Autodesk Inventor part; units mm, degrees
(part 3 of 4)
  spline S285 degree 2 poles (-3.3011, -25.9949) (-3.1963, -25.928) (-3.0357, -25.8098) knots 0 0 0 1 1 1
  line L1033 (-3.3011, -25.9949) -> (-3.1963, -25.928) construction
  line L1034 (-3.1963, -25.928) -> (-3.0357, -25.8098) construction
  spline S286 degree 2 poles (-3.0357, -25.8098) (-2.8751, -25.6805) (-2.8751, -25.5801) knots 0 0 0 1 1 1
  line L1035 (-3.0357, -25.8098) -> (-2.8751, -25.6805) construction
  line L1036 (-2.8751, -25.6805) -> (-2.8751, -25.5801) construction
  spline S287 degree 2 poles (-2.8751, -25.5801) (-2.8751, -25.4775) (-2.942, -25.4195) knots 0 0 0 1 1 1
  line L1037 (-2.8751, -25.5801) -> (-2.8751, -25.4775) construction
  line L1038 (-2.8751, -25.4775) -> (-2.942, -25.4195) construction
  spline S288 degree 2 poles (-2.942, -25.4195) (-3.0022, -25.3682) (-3.087, -25.3682) knots 0 0 0 1 1 1
  line L1039 (-2.942, -25.4195) -> (-3.0022, -25.3682) construction
  line L1040 (-3.0022, -25.3682) -> (-3.087, -25.3682) construction
  spline S289 degree 2 poles (-3.087, -25.3682) (-3.1762, -25.3682) (-3.2342, -25.4195) knots 0 0 0 1 1 1
  line L1041 (-3.087, -25.3682) -> (-3.1762, -25.3682) construction
  line L1042 (-3.1762, -25.3682) -> (-3.2342, -25.4195) construction
  spline S290 degree 2 poles (-3.2342, -25.4195) (-3.3011, -25.4775) (-3.3011, -25.5801) knots 0 0 0 1 1 1
  line L1043 (-3.2342, -25.4195) -> (-3.3011, -25.4775) construction
  line L1044 (-3.3011, -25.4775) -> (-3.3011, -25.5801) construction
  spline S291 degree 2 poles (-2.768, -27.5026) (-2.6588, -27.5026) (-2.5026, -27.3443) (-2.5026, -27.235) knots 0 0 0 1 2 2 2
  line L1045 (-2.768, -27.5026) -> (-2.6588, -27.5026) construction
  line L1046 (-2.6588, -27.5026) -> (-2.5026, -27.3443) construction
  line L1047 (-2.5026, -27.3443) -> (-2.5026, -27.235) construction
  line L1048 (-2.5026, -27.235) -> (-2.5026, -26.4343)
  spline S292 degree 2 poles (-2.5026, -26.4343) (-2.5026, -26.325) (-2.6588, -26.1667) (-2.768, -26.1667) knots 0 0 0 1 2 2 2
  line L1049 (-2.5026, -26.4343) -> (-2.5026, -26.325) construction
  line L1050 (-2.5026, -26.325) -> (-2.6588, -26.1667) construction
  line L1051 (-2.6588, -26.1667) -> (-2.768, -26.1667) construction
  line L1052 (-2.768, -26.1667) -> (-3.0357, -26.1667)
  spline S293 degree 2 poles (-3.0357, -26.1667) (-3.145, -26.1667) (-3.3011, -26.325) (-3.3011, -26.4343) knots 0 0 0 1 2 2 2
  line L1053 (-3.0357, -26.1667) -> (-3.145, -26.1667) construction
  line L1054 (-3.145, -26.1667) -> (-3.3011, -26.325) construction
  line L1055 (-3.3011, -26.325) -> (-3.3011, -26.4343) construction
  line L1056 (-3.3011, -26.4343) -> (-3.3011, -27.235)
  spline S294 degree 2 poles (-3.3011, -27.235) (-3.3011, -27.3443) (-3.145, -27.5026) (-3.0357, -27.5026) knots 0 0 0 1 2 2 2
  line L1057 (-3.3011, -27.235) -> (-3.3011, -27.3443) construction
  line L1058 (-3.3011, -27.3443) -> (-3.145, -27.5026) construction
  line L1059 (-3.145, -27.5026) -> (-3.0357, -27.5026) construction
  line L1060 (-3.0357, -27.5026) -> (-2.768, -27.5026)
  spline S295 degree 2 poles (-2.3666, -26.0619) (-2.235, -26.2024) (-2.235, -26.4343) knots 0 0 0 1 1 1
  line L1061 (-2.3666, -26.0619) -> (-2.235, -26.2024) construction
  line L1062 (-2.235, -26.2024) -> (-2.235, -26.4343) construction
  line L1063 (-2.235, -26.4343) -> (-2.235, -27.2372)
  spline S296 degree 2 poles (-2.235, -27.2372) (-2.235, -27.458) (-2.5472, -27.7703) (-2.768, -27.7703) knots 0 0 0 1 2 2 2
  line L1064 (-2.235, -27.2372) -> (-2.235, -27.458) construction
  line L1065 (-2.235, -27.458) -> (-2.5472, -27.7703) construction
  line L1066 (-2.5472, -27.7703) -> (-2.768, -27.7703) construction
  line L1067 (-2.768, -27.7703) -> (-3.0357, -27.7703)
  spline S297 degree 2 poles (-3.0357, -27.7703) (-3.2542, -27.7703) (-3.5687, -27.458) (-3.5687, -27.2372) knots 0 0 0 1 2 2 2
  line L1068 (-3.0357, -27.7703) -> (-3.2542, -27.7703) construction
  line L1069 (-3.2542, -27.7703) -> (-3.5687, -27.458) construction
  line L1070 (-3.5687, -27.458) -> (-3.5687, -27.2372) construction
  line L1071 (-3.5687, -27.2372) -> (-3.5687, -25.5801)
  spline S298 degree 2 poles (-3.5687, -25.5801) (-3.5687, -25.3549) (-3.4193, -25.221) knots 0 0 0 1 1 1
  line L1072 (-3.5687, -25.5801) -> (-3.5687, -25.3549) construction
  line L1073 (-3.5687, -25.3549) -> (-3.4193, -25.221) construction
  spline S299 degree 2 poles (-3.4193, -25.221) (-3.2832, -25.1006) (-3.0847, -25.1006) knots 0 0 0 1 1 1
  line L1074 (-3.4193, -25.221) -> (-3.2832, -25.1006) construction
  line L1075 (-3.2832, -25.1006) -> (-3.0847, -25.1006) construction
  spline S300 degree 2 poles (-3.0847, -25.1006) (-2.8907, -25.1006) (-2.7569, -25.2188) knots 0 0 0 1 1 1
  line L1076 (-3.0847, -25.1006) -> (-2.8907, -25.1006) construction
  line L1077 (-2.8907, -25.1006) -> (-2.7569, -25.2188) construction
  spline S301 degree 2 poles (-2.7569, -25.2188) (-2.6075, -25.3526) (-2.6075, -25.5779) knots 0 0 0 1 1 1
  line L1078 (-2.7569, -25.2188) -> (-2.6075, -25.3526) construction
  line L1079 (-2.6075, -25.3526) -> (-2.6075, -25.5779) construction
  spline S302 degree 2 poles (-2.6075, -25.5779) (-2.6075, -25.8031) (-2.768, -25.9102) knots 0 0 0 1 1 1
  line L1080 (-2.6075, -25.5779) -> (-2.6075, -25.8031) construction
  line L1081 (-2.6075, -25.8031) -> (-2.768, -25.9102) construction
  spline S303 degree 2 poles (-2.768, -25.9102) (-2.5093, -25.9102) (-2.3666, -26.0619) knots 0 0 0 1 1 1
  line L1082 (-2.768, -25.9102) -> (-2.5093, -25.9102) construction
  line L1083 (-2.5093, -25.9102) -> (-2.3666, -26.0619) construction
  spline S304 degree 2 poles (0.7023, -26.1689) (0.5774, -26.1689) (0.4369, -26.325) (0.4369, -26.4343) knots 0 0 0 1 2 2 2
  line L1084 (0.7023, -26.1689) -> (0.5774, -26.1689) construction
  line L1085 (0.5774, -26.1689) -> (0.4369, -26.325) construction
  line L1086 (0.4369, -26.325) -> (0.4369, -26.4343) construction
  spline S305 degree 2 poles (0.4369, -26.4343) (0.4369, -26.5436) (0.5038, -26.6194) knots 0 0 0 1 1 1
  line L1087 (0.4369, -26.4343) -> (0.4369, -26.5436) construction
  line L1088 (0.4369, -26.5436) -> (0.5038, -26.6194) construction
  spline S306 degree 2 poles (0.5038, -26.6194) (0.5774, -26.7019) (0.7023, -26.7019) knots 0 0 0 1 1 1
  line L1089 (0.5038, -26.6194) -> (0.5774, -26.7019) construction
  line L1090 (0.5774, -26.7019) -> (0.7023, -26.7019) construction
  spline S307 degree 2 poles (0.4146, -27.71) (0.3744, -27.7725) (0.3075, -27.7725) knots 0 0 0 1 1 1
  line L1091 (0.4146, -27.71) -> (0.3744, -27.7725) construction
  line L1092 (0.3744, -27.7725) -> (0.3075, -27.7725) construction
  spline S308 degree 2 poles (0.3075, -27.7725) (0.2518, -27.7725) (0.167, -27.6922) (0.167, -27.6387) knots 0 0 0 1 2 2 2
  line L1093 (0.3075, -27.7725) -> (0.2518, -27.7725) construction
  line L1094 (0.2518, -27.7725) -> (0.167, -27.6922) construction
  line L1095 (0.167, -27.6922) -> (0.167, -27.6387) construction
  spline S309 degree 2 poles (0.167, -27.6387) (0.167, -27.5985) (0.1916, -27.5628) knots 0 0 0 1 1 1
  line L1096 (0.167, -27.6387) -> (0.167, -27.5985) construction
  line L1097 (0.167, -27.5985) -> (0.1916, -27.5628) construction
  line L1098 (0.1916, -27.5628) -> (0.593, -26.9607)
  spline S310 degree 2 poles (0.593, -26.9607) (0.3923, -26.9272) (0.2741, -26.7689) knots 0 0 0 1 1 1
  line L1099 (0.593, -26.9607) -> (0.3923, -26.9272) construction
  line L1100 (0.3923, -26.9272) -> (0.2741, -26.7689) construction
  spline S311 degree 2 poles (0.2741, -26.7689) (0.1692, -26.6261) (0.1692, -26.4343) knots 0 0 0 1 1 1
  line L1101 (0.2741, -26.7689) -> (0.1692, -26.6261) construction
  line L1102 (0.1692, -26.6261) -> (0.1692, -26.4343) construction
  spline S312 degree 2 poles (0.1692, -26.4343) (0.1692, -26.218) (0.3031, -26.0685) knots 0 0 0 1 1 1
  line L1103 (0.1692, -26.4343) -> (0.1692, -26.218) construction
  line L1104 (0.1692, -26.218) -> (0.3031, -26.0685) construction
  spline S313 degree 2 poles (0.3031, -26.0685) (0.4503, -25.9013) (0.7023, -25.9013) knots 0 0 0 1 1 1
  line L1105 (0.3031, -26.0685) -> (0.4503, -25.9013) construction
  line L1106 (0.4503, -25.9013) -> (0.7023, -25.9013) construction
  line L1107 (0.7023, -25.9013) -> (1.3691, -25.9013)
  spline S314 degree 2 poles (1.3691, -25.9013) (1.503, -25.9013) (1.503, -26.0351) knots 0 0 0 1 1 1
  line L1108 (1.3691, -25.9013) -> (1.503, -25.9013) construction
  line L1109 (1.503, -25.9013) -> (1.503, -26.0351) construction
  line L1110 (1.503, -26.0351) -> (1.503, -27.6364)
  spline S315 degree 2 poles (1.503, -27.6364) (1.503, -27.7703) (1.3691, -27.7703) knots 0 0 0 1 1 1
  line L1111 (1.503, -27.6364) -> (1.503, -27.7703) construction
  line L1112 (1.503, -27.7703) -> (1.3691, -27.7703) construction
  spline S316 degree 2 poles (1.3691, -27.7703) (1.2353, -27.7703) (1.2353, -27.6364) knots 0 0 0 1 1 1
  line L1113 (1.3691, -27.7703) -> (1.2353, -27.7703) construction
  line L1114 (1.2353, -27.7703) -> (1.2353, -27.6364) construction
  spline S317 degree 2 poles (3.1846, -27.5026) (3.2627, -27.5026) (3.3719, -27.3933) (3.3719, -27.3153) knots 0 0 0 1 2 2 2
  line L1115 (3.1846, -27.5026) -> (3.2627, -27.5026) construction
  line L1116 (3.2627, -27.5026) -> (3.3719, -27.3933) construction
  line L1117 (3.3719, -27.3933) -> (3.3719, -27.3153) construction
  line L1118 (3.3719, -27.3153) -> (3.3719, -26.3563)
  spline S318 degree 2 poles (3.3719, -26.3563) (3.3719, -26.2782) (3.2627, -26.1689) (3.1846, -26.1689) knots 0 0 0 1 2 2 2
  line L1119 (3.3719, -26.3563) -> (3.3719, -26.2782) construction
  line L1120 (3.3719, -26.2782) -> (3.2627, -26.1689) construction
  line L1121 (3.2627, -26.1689) -> (3.1846, -26.1689) construction
  line L1122 (3.1846, -26.1689) -> (3.0262, -26.1689)
  spline S319 degree 2 poles (3.0262, -26.1689) (2.9482, -26.1689) (2.8389, -26.2804) (2.8389, -26.3563) knots 0 0 0 1 2 2 2
  line L1123 (3.0262, -26.1689) -> (2.9482, -26.1689) construction
  line L1124 (2.9482, -26.1689) -> (2.8389, -26.2804) construction
  line L1125 (2.8389, -26.2804) -> (2.8389, -26.3563) construction
  line L1126 (2.8389, -26.3563) -> (2.8389, -27.3153)
  spline S320 degree 2 poles (2.8389, -27.3153) (2.8389, -27.3933) (2.9482, -27.5026) (3.0262, -27.5026) knots 0 0 0 1 2 2 2
  line L1127 (2.8389, -27.3153) -> (2.8389, -27.3933) construction
  line L1128 (2.8389, -27.3933) -> (2.9482, -27.5026) construction
  line L1129 (2.9482, -27.5026) -> (3.0262, -27.5026) construction
  line L1130 (3.0262, -27.5026) -> (3.1846, -27.5026)
  spline S321 degree 2 poles (2.5713, -26.354) (2.5713, -26.1689) (2.8367, -25.9013) (3.0262, -25.9013) knots 0 0 0 1 2 2 2
  line L1131 (2.5713, -26.354) -> (2.5713, -26.1689) construction
  line L1132 (2.5713, -26.1689) -> (2.8367, -25.9013) construction
  line L1133 (2.8367, -25.9013) -> (3.0262, -25.9013) construction
  line L1134 (3.0262, -25.9013) -> (3.1846, -25.9013)
  spline S322 degree 2 poles (3.1846, -25.9013) (3.3742, -25.9013) (3.6396, -26.1667) (3.6396, -26.3563) knots 0 0 0 1 2 2 2
  line L1135 (3.1846, -25.9013) -> (3.3742, -25.9013) construction
  line L1136 (3.3742, -25.9013) -> (3.6396, -26.1667) construction
  line L1137 (3.6396, -26.1667) -> (3.6396, -26.3563) construction
  line L1138 (3.6396, -26.3563) -> (3.6396, -27.3153)
  spline S323 degree 2 poles (3.6396, -27.3153) (3.6396, -27.5049) (3.3742, -27.7703) (3.1846, -27.7703) knots 0 0 0 1 2 2 2
  line L1139 (3.6396, -27.3153) -> (3.6396, -27.5049) construction
  line L1140 (3.6396, -27.5049) -> (3.3742, -27.7703) construction
  line L1141 (3.3742, -27.7703) -> (3.1846, -27.7703) construction
  line L1142 (3.1846, -27.7703) -> (3.0262, -27.7703)
  spline S324 degree 2 poles (3.0262, -27.7703) (2.8367, -27.7703) (2.5713, -27.5071) (2.5713, -27.3175) knots 0 0 0 1 2 2 2
  line L1143 (3.0262, -27.7703) -> (2.8367, -27.7703) construction
  line L1144 (2.8367, -27.7703) -> (2.5713, -27.5071) construction
  line L1145 (2.5713, -27.5071) -> (2.5713, -27.3175) construction
  spline S325 degree 2 poles (2.3059, -27.6364) (2.3059, -27.7703) (2.172, -27.7703) knots 0 0 0 1 1 1
  line L1146 (2.3059, -27.6364) -> (2.3059, -27.7703) construction
  line L1147 (2.3059, -27.7703) -> (2.172, -27.7703) construction
  spline S326 degree 2 poles (2.172, -27.7703) (2.0382, -27.7703) (2.0382, -27.6364) knots 0 0 0 1 1 1
  line L1148 (2.172, -27.7703) -> (2.0382, -27.7703) construction
  line L1149 (2.0382, -27.7703) -> (2.0382, -27.6364) construction
  line L1150 (2.0382, -27.6364) -> (2.0382, -26.0351)
  spline S327 degree 2 poles (2.0382, -26.0351) (2.0382, -25.9013) (2.172, -25.9013) knots 0 0 0 1 1 1
  line L1151 (2.0382, -26.0351) -> (2.0382, -25.9013) construction
  line L1152 (2.0382, -25.9013) -> (2.172, -25.9013) construction
  spline S328 degree 2 poles (2.172, -25.9013) (2.3059, -25.9013) (2.3059, -26.0351) knots 0 0 0 1 1 1
  line L1153 (2.172, -25.9013) -> (2.3059, -25.9013) construction
  line L1154 (2.3059, -25.9013) -> (2.3059, -26.0351) construction
  spline S329 degree 2 poles (5.7762, -26.0351) (5.7762, -25.9013) (5.91, -25.9013) knots 0 0 0 1 1 1
  line L1155 (5.7762, -26.0351) -> (5.7762, -25.9013) construction
  line L1156 (5.7762, -25.9013) -> (5.91, -25.9013) construction
  spline S330 degree 2 poles (5.91, -25.9013) (6.0438, -25.9013) (6.0438, -26.0351) knots 0 0 0 1 1 1
  line L1157 (5.91, -25.9013) -> (6.0438, -25.9013) construction
  line L1158 (6.0438, -25.9013) -> (6.0438, -26.0351) construction
  spline S331 degree 2 poles (6.1776, -27.5026) (6.3115, -27.5026) (6.3115, -27.6364) knots 0 0 0 1 1 1
  line L1159 (6.1776, -27.5026) -> (6.3115, -27.5026) construction
  line L1160 (6.3115, -27.5026) -> (6.3115, -27.6364) construction
  line L1161 (6.3115, -27.6364) -> (6.3115, -27.9018)
  spline S332 degree 2 poles (6.3115, -27.9018) (6.3115, -28.0357) (6.1776, -28.0357) knots 0 0 0 1 1 1
  line L1162 (6.3115, -27.9018) -> (6.3115, -28.0357) construction
  line L1163 (6.3115, -28.0357) -> (6.1776, -28.0357) construction
  spline S333 degree 2 poles (6.1776, -28.0357) (6.0438, -28.0357) (6.0438, -27.9018) knots 0 0 0 1 1 1
  line L1164 (6.1776, -28.0357) -> (6.0438, -28.0357) construction
  line L1165 (6.0438, -28.0357) -> (6.0438, -27.9018) construction
  spline S334 degree 2 poles (4.7079, -27.7703) (4.4871, -27.7703) (4.1748, -27.458) (4.1748, -27.2372) knots 0 0 0 1 2 2 2
  line L1166 (4.7079, -27.7703) -> (4.4871, -27.7703) construction
  line L1167 (4.4871, -27.7703) -> (4.1748, -27.458) construction
  line L1168 (4.1748, -27.458) -> (4.1748, -27.2372) construction
  line L1169 (4.1748, -27.2372) -> (4.1748, -26.0351)
  spline S335 degree 2 poles (4.1748, -26.0351) (4.1748, -25.9013) (4.3087, -25.9013) knots 0 0 0 1 1 1
  line L1170 (4.1748, -26.0351) -> (4.1748, -25.9013) construction
  line L1171 (4.1748, -25.9013) -> (4.3087, -25.9013) construction
  spline S336 degree 2 poles (4.3087, -25.9013) (4.4425, -25.9013) (4.4425, -26.0351) knots 0 0 0 1 1 1
  line L1172 (4.3087, -25.9013) -> (4.4425, -25.9013) construction
  line L1173 (4.4425, -25.9013) -> (4.4425, -26.0351) construction
  line L1174 (4.4425, -26.0351) -> (4.4425, -27.235)
  spline S337 degree 2 poles (4.4425, -27.235) (4.4425, -27.3443) (4.6008, -27.5026) (4.7101, -27.5026) knots 0 0 0 1 2 2 2
  line L1175 (4.4425, -27.235) -> (4.4425, -27.3443) construction
  line L1176 (4.4425, -27.3443) -> (4.6008, -27.5026) construction
  line L1177 (4.6008, -27.5026) -> (4.7101, -27.5026) construction
  spline S338 degree 2 poles (4.9755, -26.0351) (4.9755, -25.9013) (5.1093, -25.9013) knots 0 0 0 1 1 1
  line L1178 (4.9755, -26.0351) -> (4.9755, -25.9013) construction
  line L1179 (4.9755, -25.9013) -> (5.1093, -25.9013) construction
  spline S339 degree 2 poles (5.1093, -25.9013) (5.2431, -25.9013) (5.2431, -26.0351) knots 0 0 0 1 1 1
  line L1180 (5.1093, -25.9013) -> (5.2431, -25.9013) construction
  line L1181 (5.2431, -25.9013) -> (5.2431, -26.0351) construction
  spline S340 degree 2 poles (-9.1062, -35.9486) (-9.3729, -35.9486) (-9.7593, -35.5677) (-9.7593, -35.2983) knots 0 0 0 1 2 2 2
  line L1182 (-9.1062, -35.9486) -> (-9.3729, -35.9486) construction
  line L1183 (-9.3729, -35.9486) -> (-9.7593, -35.5677) construction
  line L1184 (-9.7593, -35.5677) -> (-9.7593, -35.2983) construction
  line L1185 (-9.7593, -35.2983) -> (-9.7593, -34.3188)
  spline S341 degree 2 poles (-9.7593, -34.3188) (-9.7593, -34.0494) (-9.3729, -33.6685) (-9.1062, -33.6685) knots 0 0 0 1 2 2 2
  line L1186 (-9.7593, -34.3188) -> (-9.7593, -34.0494) construction
  line L1187 (-9.7593, -34.0494) -> (-9.3729, -33.6685) construction
  line L1188 (-9.3729, -33.6685) -> (-9.1062, -33.6685) construction
  line L1189 (-9.1062, -33.6685) -> (-8.6192, -33.6685)
  spline S342 degree 2 poles (-8.6192, -33.6685) (-8.4559, -33.6685) (-8.4559, -33.8317) knots 0 0 0 1 1 1
  line L1190 (-8.6192, -33.6685) -> (-8.4559, -33.6685) construction
  line L1191 (-8.4559, -33.6685) -> (-8.4559, -33.8317) construction
  spline S343 degree 2 poles (-8.4559, -33.8317) (-8.4559, -33.995) (-8.6192, -33.995) knots 0 0 0 1 1 1
  line L1192 (-8.4559, -33.8317) -> (-8.4559, -33.995) construction
  line L1193 (-8.4559, -33.995) -> (-8.6192, -33.995) construction
  line L1194 (-8.6192, -33.995) -> (-9.1062, -33.995)
  spline S344 degree 2 poles (-9.1062, -33.995) (-9.2396, -33.995) (-9.4328, -34.1882) (-9.4328, -34.3215) knots 0 0 0 1 2 2 2
  line L1195 (-9.1062, -33.995) -> (-9.2396, -33.995) construction
  line L1196 (-9.2396, -33.995) -> (-9.4328, -34.1882) construction
  line L1197 (-9.4328, -34.1882) -> (-9.4328, -34.3215) construction
  line L1198 (-9.4328, -34.3215) -> (-9.4328, -35.2956)
  spline S345 degree 2 poles (-9.4328, -35.2956) (-9.4328, -35.4289) (-9.2396, -35.6221) (-9.1062, -35.6221) knots 0 0 0 1 2 2 2
  line L1199 (-9.4328, -35.2956) -> (-9.4328, -35.4289) construction
  line L1200 (-9.4328, -35.4289) -> (-9.2396, -35.6221) construction
  line L1201 (-9.2396, -35.6221) -> (-9.1062, -35.6221) construction
  line L1202 (-9.1062, -35.6221) -> (-8.6192, -35.6221)
  spline S346 degree 2 poles (-8.6192, -35.6221) (-8.4559, -35.6221) (-8.4559, -35.7854) knots 0 0 0 1 1 1
  line L1203 (-8.6192, -35.6221) -> (-8.4559, -35.6221) construction
  line L1204 (-8.4559, -35.6221) -> (-8.4559, -35.7854) construction
  spline S347 degree 2 poles (-8.4559, -35.7854) (-8.4559, -35.9486) (-8.6192, -35.9486) knots 0 0 0 1 1 1
  line L1205 (-8.4559, -35.7854) -> (-8.4559, -35.9486) construction
  line L1206 (-8.4559, -35.9486) -> (-8.6192, -35.9486) construction
  line L1207 (-8.6192, -35.9486) -> (-9.1062, -35.9486)
  spline S348 degree 2 poles (-3.0954, -34.8826) (-3.3631, -34.8826) (-3.3631, -34.6149) knots 0 0 0 1 1 1
  line L1208 (-3.0954, -34.8826) -> (-3.3631, -34.8826) construction
  line L1209 (-3.3631, -34.8826) -> (-3.3631, -34.6149) construction
  spline S349 degree 2 poles (-3.3631, -34.6149) (-3.3631, -34.3473) (-3.0954, -34.3473) knots 0 0 0 1 1 1
  line L1210 (-3.3631, -34.6149) -> (-3.3631, -34.3473) construction
  line L1211 (-3.3631, -34.3473) -> (-3.0954, -34.3473) construction
  line L1212 (-3.0954, -34.3473) -> (-0.9588, -34.3473)
  spline S350 degree 2 poles (-0.9588, -34.3473) (-0.6957, -34.3473) (-0.6957, -34.6149) knots 0 0 0 1 1 1
  line L1213 (-0.9588, -34.3473) -> (-0.6957, -34.3473) construction
  line L1214 (-0.6957, -34.3473) -> (-0.6957, -34.6149) construction
  spline S351 degree 2 poles (-0.6957, -34.6149) (-0.6957, -34.8826) (-0.9588, -34.8826) knots 0 0 0 1 1 1
  line L1215 (-0.6957, -34.6149) -> (-0.6957, -34.8826) construction
  line L1216 (-0.6957, -34.8826) -> (-0.9588, -34.8826) construction
  line L1217 (-0.9588, -34.8826) -> (-3.0954, -34.8826)
  spline S352 degree 2 poles (-11.6176, -39.3084) (-11.6176, -39.1745) (-11.4838, -39.1745) knots 0 0 0 1 1 1
  line L1218 (-11.6176, -39.3084) -> (-11.6176, -39.1745) construction
  line L1219 (-11.6176, -39.1745) -> (-11.4838, -39.1745) construction
  spline S353 degree 2 poles (-11.4838, -39.1745) (-11.35, -39.1745) (-11.35, -39.3084) knots 0 0 0 1 1 1
  line L1220 (-11.4838, -39.1745) -> (-11.35, -39.1745) construction
  line L1221 (-11.35, -39.1745) -> (-11.35, -39.3084) construction
  line L1222 (-11.35, -39.3084) -> (-11.35, -40.9097)
  spline S354 degree 2 poles (-11.35, -40.9097) (-11.35, -41.0435) (-11.4838, -41.0435) knots 0 0 0 1 1 1
  line L1223 (-11.35, -40.9097) -> (-11.35, -41.0435) construction
  line L1224 (-11.35, -41.0435) -> (-11.4838, -41.0435) construction
  spline S355 degree 2 poles (-11.4838, -41.0435) (-11.6176, -41.0435) (-11.6176, -40.9097) knots 0 0 0 1 1 1
  line L1225 (-11.4838, -41.0435) -> (-11.6176, -41.0435) construction
  line L1226 (-11.6176, -41.0435) -> (-11.6176, -40.9097) construction
  spline S356 degree 2 poles (-12.416, -40.9097) (-12.416, -41.0435) (-12.5499, -41.0435) knots 0 0 0 1 1 1
  line L1227 (-12.416, -40.9097) -> (-12.416, -41.0435) construction
  line L1228 (-12.416, -41.0435) -> (-12.5499, -41.0435) construction
  spline S357 degree 2 poles (-12.5499, -41.0435) (-12.6837, -41.0435) (-12.6837, -40.9097) knots 0 0 0 1 1 1
  line L1229 (-12.5499, -41.0435) -> (-12.6837, -41.0435) construction
  line L1230 (-12.6837, -41.0435) -> (-12.6837, -40.9097) construction
  line L1231 (-12.6837, -40.9097) -> (-12.6837, -39.3084)
  spline S358 degree 2 poles (-12.6837, -39.3084) (-12.6837, -39.1745) (-12.5499, -39.1745) knots 0 0 0 1 1 1
  line L1232 (-12.6837, -39.3084) -> (-12.6837, -39.1745) construction
  line L1233 (-12.6837, -39.1745) -> (-12.5499, -39.1745) construction
  spline S359 degree 2 poles (-12.5499, -39.1745) (-12.416, -39.1745) (-12.416, -39.3084) knots 0 0 0 1 1 1
  line L1234 (-12.5499, -39.1745) -> (-12.416, -39.1745) construction
  line L1235 (-12.416, -39.1745) -> (-12.416, -39.3084) construction
  spline S360 degree 2 poles (-5.8769, -41.0435) (-6.0107, -41.0435) (-6.0107, -40.9097) knots 0 0 0 1 1 1
  line L1236 (-5.8769, -41.0435) -> (-6.0107, -41.0435) construction
  line L1237 (-6.0107, -41.0435) -> (-6.0107, -40.9097) construction
  spline S361 degree 2 poles (-6.818, -40.9521) (-6.847, -41.0435) (-6.9362, -41.0435) knots 0 0 0 1 1 1
  line L1238 (-6.818, -40.9521) -> (-6.847, -41.0435) construction
  line L1239 (-6.847, -41.0435) -> (-6.9362, -41.0435) construction
  spline S362 degree 2 poles (-6.9362, -41.0435) (-7.0767, -41.0435) (-7.0767, -40.9164) knots 0 0 0 1 1 1
  line L1240 (-6.9362, -41.0435) -> (-7.0767, -41.0435) construction
  line L1241 (-7.0767, -41.0435) -> (-7.0767, -40.9164) construction
  spline S363 degree 2 poles (-7.0767, -40.9164) (-7.0767, -40.8919) (-7.0678, -40.8673) knots 0 0 0 1 1 1
  line L1242 (-7.0767, -40.9164) -> (-7.0767, -40.8919) construction
  line L1243 (-7.0767, -40.8919) -> (-7.0678, -40.8673) construction
  line L1244 (-7.0678, -40.8673) -> (-6.5392, -39.266)
  spline S364 degree 2 poles (-6.5392, -39.266) (-6.5103, -39.1745) (-6.4144, -39.1745) knots 0 0 0 1 1 1
  line L1245 (-6.5392, -39.266) -> (-6.5103, -39.1745) construction
  line L1246 (-6.5103, -39.1745) -> (-6.4144, -39.1745) construction
  line L1247 (-6.4144, -39.1745) -> (-5.8769, -39.1745)
  spline S365 degree 2 poles (-5.8769, -39.1745) (-5.743, -39.1745) (-5.743, -39.3084) knots 0 0 0 1 1 1
  line L1248 (-5.8769, -39.1745) -> (-5.743, -39.1745) construction
  line L1249 (-5.743, -39.1745) -> (-5.743, -39.3084) construction
  line L1250 (-5.743, -39.3084) -> (-5.743, -40.9097)
  spline S366 degree 2 poles (-5.743, -40.9097) (-5.743, -41.0435) (-5.8769, -41.0435) knots 0 0 0 1 1 1
  line L1251 (-5.743, -40.9097) -> (-5.743, -41.0435) construction
  line L1252 (-5.743, -41.0435) -> (-5.8769, -41.0435) construction
  spline S367 degree 2 poles (1.1976, -39.3084) (1.1976, -39.1745) (1.3314, -39.1745) knots 0 0 0 1 1 1
  line L1253 (1.1976, -39.3084) -> (1.1976, -39.1745) construction
  line L1254 (1.1976, -39.1745) -> (1.3314, -39.1745) construction
  spline S368 degree 2 poles (1.3314, -39.1745) (1.4652, -39.1745) (1.4652, -39.3084) knots 0 0 0 1 1 1
  line L1255 (1.3314, -39.1745) -> (1.4652, -39.1745) construction
  line L1256 (1.4652, -39.1745) -> (1.4652, -39.3084) construction
  line L1257 (1.4652, -39.3084) -> (1.4652, -40.9097)
  spline S369 degree 2 poles (1.4652, -40.9097) (1.4652, -41.0435) (1.3314, -41.0435) knots 0 0 0 1 1 1
  line L1258 (1.4652, -40.9097) -> (1.4652, -41.0435) construction
  line L1259 (1.4652, -41.0435) -> (1.3314, -41.0435) construction
  spline S370 degree 2 poles (1.3314, -41.0435) (1.1976, -41.0435) (1.1976, -40.9097) knots 0 0 0 1 1 1
  line L1260 (1.3314, -41.0435) -> (1.1976, -41.0435) construction
  line L1261 (1.1976, -41.0435) -> (1.1976, -40.9097) construction
  spline S371 degree 2 poles (0.3992, -40.9097) (0.3992, -41.0435) (0.2653, -41.0435) knots 0 0 0 1 1 1
  line L1262 (0.3992, -40.9097) -> (0.3992, -41.0435) construction
  line L1263 (0.3992, -41.0435) -> (0.2653, -41.0435) construction
  spline S372 degree 2 poles (0.2653, -41.0435) (0.1315, -41.0435) (0.1315, -40.9097) knots 0 0 0 1 1 1
  line L1264 (0.2653, -41.0435) -> (0.1315, -41.0435) construction
  line L1265 (0.1315, -41.0435) -> (0.1315, -40.9097) construction
  line L1266 (0.1315, -40.9097) -> (0.1315, -39.3084)
  spline S373 degree 2 poles (0.1315, -39.3084) (0.1315, -39.1745) (0.2653, -39.1745) knots 0 0 0 1 1 1
  line L1267 (0.1315, -39.3084) -> (0.1315, -39.1745) construction
  line L1268 (0.1315, -39.1745) -> (0.2653, -39.1745) construction
  spline S374 degree 2 poles (0.2653, -39.1745) (0.3992, -39.1745) (0.3992, -39.3084) knots 0 0 0 1 1 1
  line L1269 (0.2653, -39.1745) -> (0.3992, -39.1745) construction
  line L1270 (0.3992, -39.1745) -> (0.3992, -39.3084) construction
  spline S375 degree 2 poles (6.5391, -40.7759) (6.6484, -40.7759) (6.8045, -40.6175) (6.8045, -40.5083) knots 0 0 0 1 2 2 2
  line L1271 (6.5391, -40.7759) -> (6.6484, -40.7759) construction
  line L1272 (6.6484, -40.7759) -> (6.8045, -40.6175) construction
  line L1273 (6.8045, -40.6175) -> (6.8045, -40.5083) construction
  line L1274 (6.8045, -40.5083) -> (6.8045, -39.7098)
  spline S376 degree 2 poles (6.8045, -39.7098) (6.8045, -39.6005) (6.6484, -39.4422) (6.5391, -39.4422) knots 0 0 0 1 2 2 2
  line L1275 (6.8045, -39.7098) -> (6.8045, -39.6005) construction
  line L1276 (6.8045, -39.6005) -> (6.6484, -39.4422) construction
  line L1277 (6.6484, -39.4422) -> (6.5391, -39.4422) construction
  spline S377 degree 2 poles (6.0061, -41.7104) (6.0061, -41.8442) (5.8723, -41.8442) knots 0 0 0 1 1 1
  line L1278 (6.0061, -41.7104) -> (6.0061, -41.8442) construction
  line L1279 (6.0061, -41.8442) -> (5.8723, -41.8442) construction
  spline S378 degree 2 poles (5.8723, -41.8442) (5.7385, -41.8442) (5.7385, -41.7104) knots 0 0 0 1 1 1
  line L1280 (5.8723, -41.8442) -> (5.7385, -41.8442) construction
  line L1281 (5.7385, -41.8442) -> (5.7385, -41.7104) construction
  line L1282 (5.7385, -41.7104) -> (5.7385, -39.3084)
  spline S379 degree 2 poles (5.7385, -39.3084) (5.7385, -39.1745) (5.8723, -39.1745) knots 0 0 0 1 1 1
  line L1283 (5.7385, -39.3084) -> (5.7385, -39.1745) construction
  line L1284 (5.7385, -39.1745) -> (5.8723, -39.1745) construction
  line L1285 (5.8723, -39.1745) -> (6.5391, -39.1745)
  spline S380 degree 2 poles (6.5391, -39.1745) (6.7599, -39.1745) (7.0722, -39.4868) (7.0722, -39.7076) knots 0 0 0 1 2 2 2
  line L1286 (6.5391, -39.1745) -> (6.7599, -39.1745) construction
  line L1287 (6.7599, -39.1745) -> (7.0722, -39.4868) construction
  line L1288 (7.0722, -39.4868) -> (7.0722, -39.7076) construction
  line L1289 (7.0722, -39.7076) -> (7.0722, -40.5105)
  spline S381 degree 2 poles (7.0722, -40.5105) (7.0722, -40.7313) (6.7599, -41.0435) (6.5391, -41.0435) knots 0 0 0 1 2 2 2
  line L1290 (7.0722, -40.5105) -> (7.0722, -40.7313) construction
  line L1291 (7.0722, -40.7313) -> (6.7599, -41.0435) construction
  line L1292 (6.7599, -41.0435) -> (6.5391, -41.0435) construction
  spline S382 degree 2 poles (8.4081, -40.7759) (8.5174, -40.7759) (8.6735, -40.6175) (8.6735, -40.5083) knots 0 0 0 1 2 2 2
  line L1293 (8.4081, -40.7759) -> (8.5174, -40.7759) construction
  line L1294 (8.5174, -40.7759) -> (8.6735, -40.6175) construction
  line L1295 (8.6735, -40.6175) -> (8.6735, -40.5083) construction
  spline S383 degree 2 poles (8.1405, -39.4422) (8.0312, -39.4422) (7.8751, -39.6005) (7.8751, -39.7098) knots 0 0 0 1 2 2 2
  line L1296 (8.1405, -39.4422) -> (8.0312, -39.4422) construction
  line L1297 (8.0312, -39.4422) -> (7.8751, -39.6005) construction
  line L1298 (7.8751, -39.6005) -> (7.8751, -39.7098) construction
  line L1299 (7.8751, -39.7098) -> (7.8751, -40.5083)
  spline S384 degree 2 poles (7.8751, -40.5083) (7.8751, -40.6175) (8.0312, -40.7759) (8.1405, -40.7759) knots 0 0 0 1 2 2 2
  line L1300 (7.8751, -40.5083) -> (7.8751, -40.6175) construction
  line L1301 (7.8751, -40.6175) -> (8.0312, -40.7759) construction
  line L1302 (8.0312, -40.7759) -> (8.1405, -40.7759) construction
  line L1303 (8.1405, -40.7759) -> (8.4081, -40.7759)
  line L1304 (8.4081, -41.0435) -> (8.1405, -41.0435)
  spline S385 degree 2 poles (8.1405, -41.0435) (7.9219, -41.0435) (7.6074, -40.7313) (7.6074, -40.5105) knots 0 0 0 1 2 2 2
  line L1305 (8.1405, -41.0435) -> (7.9219, -41.0435) construction
  line L1306 (7.9219, -41.0435) -> (7.6074, -40.7313) construction
  line L1307 (7.6074, -40.7313) -> (7.6074, -40.5105) construction
  line L1308 (7.6074, -40.5105) -> (7.6074, -39.7076)
  spline S386 degree 2 poles (7.6074, -39.7076) (7.6074, -39.4868) (7.9219, -39.1745) (8.1405, -39.1745) knots 0 0 0 1 2 2 2
  line L1309 (7.6074, -39.7076) -> (7.6074, -39.4868) construction
  line L1310 (7.6074, -39.4868) -> (7.9219, -39.1745) construction
  line L1311 (7.9219, -39.1745) -> (8.1405, -39.1745) construction
  line L1312 (8.1405, -39.1745) -> (8.8073, -39.1745)
  spline S387 degree 2 poles (8.8073, -39.1745) (8.9412, -39.1745) (8.9412, -39.3084) knots 0 0 0 1 1 1
  line L1313 (8.8073, -39.1745) -> (8.9412, -39.1745) construction
  line L1314 (8.9412, -39.1745) -> (8.9412, -39.3084) construction
  line L1315 (8.9412, -39.3084) -> (8.9412, -40.506)
  spline S388 degree 2 poles (8.9412, -40.506) (8.9412, -40.7068) (9.1285, -40.787) knots 0 0 0 1 1 1
  line L1316 (8.9412, -40.506) -> (8.9412, -40.7068) construction
  line L1317 (8.9412, -40.7068) -> (9.1285, -40.787) construction
  spline S389 degree 2 poles (9.1285, -40.787) (9.211, -40.8205) (9.211, -40.9052) knots 0 0 0 1 1 1
  line L1318 (9.1285, -40.787) -> (9.211, -40.8205) construction
  line L1319 (9.211, -40.8205) -> (9.211, -40.9052) construction
  spline S390 degree 2 poles (9.211, -40.9052) (9.211, -40.961) (9.1352, -41.0458) (9.0794, -41.0458) knots 0 0 0 1 2 2 2
  line L1320 (9.211, -40.9052) -> (9.211, -40.961) construction
  line L1321 (9.211, -40.961) -> (9.1352, -41.0458) construction
  line L1322 (9.1352, -41.0458) -> (9.0794, -41.0458) construction
  spline S391 degree 2 poles (9.0794, -41.0458) (9.0504, -41.0458) (9.0214, -41.0324) knots 0 0 0 1 1 1
  line L1323 (9.0794, -41.0458) -> (9.0504, -41.0458) construction
  line L1324 (9.0504, -41.0458) -> (9.0214, -41.0324) construction
  spline S392 degree 2 poles (9.0214, -41.0324) (8.8876, -40.9744) (8.8051, -40.8673) knots 0 0 0 1 1 1
  line L1325 (9.0214, -41.0324) -> (8.8876, -40.9744) construction
  line L1326 (8.8876, -40.9744) -> (8.8051, -40.8673) construction
  spline S393 degree 2 poles (8.8051, -40.8673) (8.6445, -41.0435) (8.4081, -41.0435) knots 0 0 0 1 1 1
  line L1327 (8.8051, -40.8673) -> (8.6445, -41.0435) construction
  line L1328 (8.6445, -41.0435) -> (8.4081, -41.0435) construction
  line L1329 (9.7441, -38.8534) -> (9.7441, -39.2682)
  spline S394 degree 2 poles (9.7441, -39.2682) (9.8489, -39.2013) (10.0095, -39.0831) knots 0 0 0 1 1 1
  line L1330 (9.7441, -39.2682) -> (9.8489, -39.2013) construction
  line L1331 (9.8489, -39.2013) -> (10.0095, -39.0831) construction
  spline S395 degree 2 poles (10.0095, -39.0831) (10.17, -38.9537) (10.17, -38.8534) knots 0 0 0 1 1 1
  line L1332 (10.0095, -39.0831) -> (10.17, -38.9537) construction
  line L1333 (10.17, -38.9537) -> (10.17, -38.8534) construction
  spline S396 degree 2 poles (10.17, -38.8534) (10.17, -38.7508) (10.1031, -38.6928) knots 0 0 0 1 1 1
  line L1334 (10.17, -38.8534) -> (10.17, -38.7508) construction
  line L1335 (10.17, -38.7508) -> (10.1031, -38.6928) construction
  spline S397 degree 2 poles (10.1031, -38.6928) (10.0429, -38.6415) (9.9582, -38.6415) knots 0 0 0 1 1 1
  line L1336 (10.1031, -38.6928) -> (10.0429, -38.6415) construction
  line L1337 (10.0429, -38.6415) -> (9.9582, -38.6415) construction
  spline S398 degree 2 poles (9.9582, -38.6415) (9.869, -38.6415) (9.811, -38.6928) knots 0 0 0 1 1 1
  line L1338 (9.9582, -38.6415) -> (9.869, -38.6415) construction
  line L1339 (9.869, -38.6415) -> (9.811, -38.6928) construction
  spline S399 degree 2 poles (9.811, -38.6928) (9.7441, -38.7508) (9.7441, -38.8534) knots 0 0 0 1 1 1
  line L1340 (9.811, -38.6928) -> (9.7441, -38.7508) construction
  line L1341 (9.7441, -38.7508) -> (9.7441, -38.8534) construction
  spline S400 degree 2 poles (10.2771, -40.7759) (10.3864, -40.7759) (10.5425, -40.6175) (10.5425, -40.5083) knots 0 0 0 1 2 2 2
  line L1342 (10.2771, -40.7759) -> (10.3864, -40.7759) construction
  line L1343 (10.3864, -40.7759) -> (10.5425, -40.6175) construction
  line L1344 (10.5425, -40.6175) -> (10.5425, -40.5083) construction
  line L1345 (10.5425, -40.5083) -> (10.5425, -39.7076)
  spline S401 degree 2 poles (10.5425, -39.7076) (10.5425, -39.5983) (10.3864, -39.44) (10.2771, -39.44) knots 0 0 0 1 2 2 2
  line L1346 (10.5425, -39.7076) -> (10.5425, -39.5983) construction
  line L1347 (10.5425, -39.5983) -> (10.3864, -39.44) construction
  line L1348 (10.3864, -39.44) -> (10.2771, -39.44) construction
  line L1349 (10.2771, -39.44) -> (10.0095, -39.44)
  spline S402 degree 2 poles (10.0095, -39.44) (9.9002, -39.44) (9.7441, -39.5983) (9.7441, -39.7076) knots 0 0 0 1 2 2 2
  line L1350 (10.0095, -39.44) -> (9.9002, -39.44) construction
  line L1351 (9.9002, -39.44) -> (9.7441, -39.5983) construction
  line L1352 (9.7441, -39.5983) -> (9.7441, -39.7076) construction
  line L1353 (9.7441, -39.7076) -> (9.7441, -40.5083)
  spline S403 degree 2 poles (9.7441, -40.5083) (9.7441, -40.6175) (9.9002, -40.7759) (10.0095, -40.7759) knots 0 0 0 1 2 2 2
  line L1354 (9.7441, -40.5083) -> (9.7441, -40.6175) construction
  line L1355 (9.7441, -40.6175) -> (9.9002, -40.7759) construction
  line L1356 (9.9002, -40.7759) -> (10.0095, -40.7759) construction
  line L1357 (10.0095, -40.7759) -> (10.2771, -40.7759)
  spline S404 degree 2 poles (10.6785, -39.3351) (10.8101, -39.4756) (10.8101, -39.7076) knots 0 0 0 1 1 1
  line L1358 (10.6785, -39.3351) -> (10.8101, -39.4756) construction
  line L1359 (10.8101, -39.4756) -> (10.8101, -39.7076) construction
  line L1360 (10.8101, -39.7076) -> (10.8101, -40.5105)
  spline S405 degree 2 poles (10.8101, -40.5105) (10.8101, -40.7313) (10.4979, -41.0435) (10.2771, -41.0435) knots 0 0 0 1 2 2 2
  line L1361 (10.8101, -40.5105) -> (10.8101, -40.7313) construction
  line L1362 (10.8101, -40.7313) -> (10.4979, -41.0435) construction
  line L1363 (10.4979, -41.0435) -> (10.2771, -41.0435) construction
  line L1364 (10.2771, -41.0435) -> (10.0095, -41.0435)
  spline S406 degree 2 poles (10.0095, -41.0435) (9.7909, -41.0435) (9.4764, -40.7313) (9.4764, -40.5105) knots 0 0 0 1 2 2 2
  line L1365 (10.0095, -41.0435) -> (9.7909, -41.0435) construction
  line L1366 (9.7909, -41.0435) -> (9.4764, -40.7313) construction
  line L1367 (9.4764, -40.7313) -> (9.4764, -40.5105) construction
  line L1368 (9.4764, -40.5105) -> (9.4764, -38.8534)
  spline S407 degree 2 poles (9.4764, -38.8534) (9.4764, -38.6281) (9.6259, -38.4943) knots 0 0 0 1 1 1
  line L1369 (9.4764, -38.8534) -> (9.4764, -38.6281) construction
  line L1370 (9.4764, -38.6281) -> (9.6259, -38.4943) construction
  spline S408 degree 2 poles (9.6259, -38.4943) (9.7619, -38.3739) (9.9604, -38.3739) knots 0 0 0 1 1 1
  line L1371 (9.6259, -38.4943) -> (9.7619, -38.3739) construction
  line L1372 (9.7619, -38.3739) -> (9.9604, -38.3739) construction
  spline S409 degree 2 poles (9.9604, -38.3739) (10.1544, -38.3739) (10.2882, -38.4921) knots 0 0 0 1 1 1
  line L1373 (9.9604, -38.3739) -> (10.1544, -38.3739) construction
  line L1374 (10.1544, -38.3739) -> (10.2882, -38.4921) construction
  spline S410 degree 2 poles (10.2882, -38.4921) (10.4377, -38.6259) (10.4377, -38.8512) knots 0 0 0 1 1 1
  line L1375 (10.2882, -38.4921) -> (10.4377, -38.6259) construction
  line L1376 (10.4377, -38.6259) -> (10.4377, -38.8512) construction
  spline S411 degree 2 poles (10.4377, -38.8512) (10.4377, -39.0764) (10.2771, -39.1835) knots 0 0 0 1 1 1
  line L1377 (10.4377, -38.8512) -> (10.4377, -39.0764) construction
  line L1378 (10.4377, -39.0764) -> (10.2771, -39.1835) construction
  spline S412 degree 2 poles (10.2771, -39.1835) (10.5358, -39.1835) (10.6785, -39.3351) knots 0 0 0 1 1 1
  line L1379 (10.2771, -39.1835) -> (10.5358, -39.1835) construction
  line L1380 (10.5358, -39.1835) -> (10.6785, -39.3351) construction
  spline S413 degree 2 poles (13.3482, -40.7759) (13.482, -40.7759) (13.482, -40.9097) knots 0 0 0 1 1 1
  line L1381 (13.3482, -40.7759) -> (13.482, -40.7759) construction
  line L1382 (13.482, -40.7759) -> (13.482, -40.9097) construction
  spline S414 degree 2 poles (13.482, -40.9097) (13.482, -41.0435) (13.3482, -41.0435) knots 0 0 0 1 1 1
  line L1383 (13.482, -40.9097) -> (13.482, -41.0435) construction
  line L1384 (13.482, -41.0435) -> (13.3482, -41.0435) construction
  spline S415 degree 2 poles (13.3482, -41.0435) (13.2144, -41.0435) (13.2144, -40.9097) knots 0 0 0 1 1 1
  line L1385 (13.3482, -41.0435) -> (13.2144, -41.0435) construction
  line L1386 (13.2144, -41.0435) -> (13.2144, -40.9097) construction
  spline S416 degree 2 poles (13.2144, -40.9097) (13.2144, -40.7759) (13.3482, -40.7759) knots 0 0 0 1 1 1
  line L1387 (13.2144, -40.9097) -> (13.2144, -40.7759) construction
  line L1388 (13.2144, -40.7759) -> (13.3482, -40.7759) construction
  spline S417 degree 2 poles (-5.1574, 29.3464) (-5.0326, 29.3464) (-4.959, 29.4289) knots 0 0 0 1 1 1
  line L1389 (-5.1574, 29.3464) -> (-5.0326, 29.3464) construction
  line L1390 (-5.0326, 29.3464) -> (-4.959, 29.4289) construction
  spline S418 degree 2 poles (-4.959, 29.4289) (-4.892, 29.5047) (-4.892, 29.614) knots 0 0 0 1 1 1
  line L1391 (-4.959, 29.4289) -> (-4.892, 29.5047) construction
  line L1392 (-4.892, 29.5047) -> (-4.892, 29.614) construction
  spline S419 degree 2 poles (-4.892, 29.614) (-4.892, 29.7233) (-4.959, 29.7969) knots 0 0 0 1 1 1
  line L1393 (-4.892, 29.614) -> (-4.892, 29.7233) construction
  line L1394 (-4.892, 29.7233) -> (-4.959, 29.7969) construction
  spline S420 degree 2 poles (-4.959, 29.7969) (-5.0326, 29.8794) (-5.1574, 29.8794) knots 0 0 0 1 1 1
  line L1395 (-4.959, 29.7969) -> (-5.0326, 29.8794) construction
  line L1396 (-5.0326, 29.8794) -> (-5.1574, 29.8794) construction
  spline S421 degree 2 poles (-5.1574, 30.147) (-4.9032, 30.147) (-4.7582, 29.9798) knots 0 0 0 1 1 1
  line L1397 (-5.1574, 30.147) -> (-4.9032, 30.147) construction
  line L1398 (-4.9032, 30.147) -> (-4.7582, 29.9798) construction
  spline S422 degree 2 poles (-4.7582, 29.9798) (-4.6244, 29.8303) (-4.6244, 29.614) knots 0 0 0 1 1 1
  line L1399 (-4.7582, 29.9798) -> (-4.6244, 29.8303) construction
  line L1400 (-4.6244, 29.8303) -> (-4.6244, 29.614) construction
  spline S423 degree 2 poles (-4.6244, 29.614) (-4.6244, 29.3977) (-4.7582, 29.2438) knots 0 0 0 1 1 1
  line L1401 (-4.6244, 29.614) -> (-4.6244, 29.3977) construction
  line L1402 (-4.6244, 29.3977) -> (-4.7582, 29.2438) construction
  spline S424 degree 2 poles (-4.7582, 29.2438) (-4.9054, 29.0787) (-5.1574, 29.0787) knots 0 0 0 1 1 1
  line L1403 (-4.7582, 29.2438) -> (-4.9054, 29.0787) construction
  line L1404 (-4.9054, 29.0787) -> (-5.1574, 29.0787) construction
  line L1405 (-5.1574, 29.0787) -> (-5.8243, 29.0787)
  spline S425 degree 2 poles (-5.8243, 29.0787) (-5.9581, 29.0787) (-5.9581, 29.2126) knots 0 0 0 1 1 1
  line L1406 (-5.8243, 29.0787) -> (-5.9581, 29.0787) construction
  line L1407 (-5.9581, 29.0787) -> (-5.9581, 29.2126) construction
  line L1408 (-5.9581, 29.2126) -> (-5.9581, 30.8139)
  spline S426 degree 2 poles (-5.9581, 30.8139) (-5.9581, 30.9477) (-5.8243, 30.9477) knots 0 0 0 1 1 1
  line L1409 (-5.9581, 30.8139) -> (-5.9581, 30.9477) construction
  line L1410 (-5.9581, 30.9477) -> (-5.8243, 30.9477) construction
  spline S427 degree 2 poles (-5.8243, 30.9477) (-5.6905, 30.9477) (-5.6905, 30.8139) knots 0 0 0 1 1 1
  line L1411 (-5.8243, 30.9477) -> (-5.6905, 30.9477) construction
  line L1412 (-5.6905, 30.9477) -> (-5.6905, 30.8139) construction
  line L1413 (-11.1636, 31.2689) -> (-11.1636, 30.854)
  spline S428 degree 2 poles (-11.1636, 30.854) (-11.0588, 30.921) (-10.8982, 31.0392) knots 0 0 0 1 1 1
  line L1414 (-11.1636, 30.854) -> (-11.0588, 30.921) construction
  line L1415 (-11.0588, 30.921) -> (-10.8982, 31.0392) construction
  spline S429 degree 2 poles (-10.8982, 31.0392) (-10.7376, 31.1685) (-10.7376, 31.2689) knots 0 0 0 1 1 1
  line L1416 (-10.8982, 31.0392) -> (-10.7376, 31.1685) construction
  line L1417 (-10.7376, 31.1685) -> (-10.7376, 31.2689) construction
  spline S430 degree 2 poles (-10.7376, 31.2689) (-10.7376, 31.3715) (-10.8045, 31.4295) knots 0 0 0 1 1 1
  line L1418 (-10.7376, 31.2689) -> (-10.7376, 31.3715) construction
  line L1419 (-10.7376, 31.3715) -> (-10.8045, 31.4295) construction
  spline S431 degree 2 poles (-10.8045, 31.4295) (-10.8647, 31.4808) (-10.9495, 31.4808) knots 0 0 0 1 1 1
  line L1420 (-10.8045, 31.4295) -> (-10.8647, 31.4808) construction
  line L1421 (-10.8647, 31.4808) -> (-10.9495, 31.4808) construction
  spline S432 degree 2 poles (-10.9495, 31.4808) (-11.0387, 31.4808) (-11.0967, 31.4295) knots 0 0 0 1 1 1
  line L1422 (-10.9495, 31.4808) -> (-11.0387, 31.4808) construction
  line L1423 (-11.0387, 31.4808) -> (-11.0967, 31.4295) construction
  spline S433 degree 2 poles (-11.0967, 31.4295) (-11.1636, 31.3715) (-11.1636, 31.2689) knots 0 0 0 1 1 1
  line L1424 (-11.0967, 31.4295) -> (-11.1636, 31.3715) construction
  line L1425 (-11.1636, 31.3715) -> (-11.1636, 31.2689) construction
  spline S434 degree 2 poles (-10.6306, 29.3464) (-10.5213, 29.3464) (-10.3652, 29.5047) (-10.3652, 29.614) knots 0 0 0 1 2 2 2
  line L1426 (-10.6306, 29.3464) -> (-10.5213, 29.3464) construction
  line L1427 (-10.5213, 29.3464) -> (-10.3652, 29.5047) construction
  line L1428 (-10.3652, 29.5047) -> (-10.3652, 29.614) construction
  line L1429 (-10.3652, 29.614) -> (-10.3652, 30.4147)
  spline S435 degree 2 poles (-10.3652, 30.4147) (-10.3652, 30.524) (-10.5213, 30.6823) (-10.6306, 30.6823) knots 0 0 0 1 2 2 2
  line L1430 (-10.3652, 30.4147) -> (-10.3652, 30.524) construction
  line L1431 (-10.3652, 30.524) -> (-10.5213, 30.6823) construction
  line L1432 (-10.5213, 30.6823) -> (-10.6306, 30.6823) construction
  line L1433 (-10.6306, 30.6823) -> (-10.8982, 30.6823)
  spline S436 degree 2 poles (-10.8982, 30.6823) (-11.0075, 30.6823) (-11.1636, 30.524) (-11.1636, 30.4147) knots 0 0 0 1 2 2 2
  line L1434 (-10.8982, 30.6823) -> (-11.0075, 30.6823) construction
  line L1435 (-11.0075, 30.6823) -> (-11.1636, 30.524) construction
  line L1436 (-11.1636, 30.524) -> (-11.1636, 30.4147) construction
  line L1437 (-11.1636, 30.4147) -> (-11.1636, 29.614)
  spline S437 degree 2 poles (-11.1636, 29.614) (-11.1636, 29.5047) (-11.0075, 29.3464) (-10.8982, 29.3464) knots 0 0 0 1 2 2 2
  line L1438 (-11.1636, 29.614) -> (-11.1636, 29.5047) construction
  line L1439 (-11.1636, 29.5047) -> (-11.0075, 29.3464) construction
  line L1440 (-11.0075, 29.3464) -> (-10.8982, 29.3464) construction
  line L1441 (-10.8982, 29.3464) -> (-10.6306, 29.3464)
  spline S438 degree 2 poles (-10.2291, 30.7871) (-10.0975, 30.6466) (-10.0975, 30.4147) knots 0 0 0 1 1 1
  line L1442 (-10.2291, 30.7871) -> (-10.0975, 30.6466) construction
  line L1443 (-10.0975, 30.6466) -> (-10.0975, 30.4147) construction
  line L1444 (-10.0975, 30.4147) -> (-10.0975, 29.6118)
  spline S439 degree 2 poles (-10.0975, 29.6118) (-10.0975, 29.391) (-10.4098, 29.0787) (-10.6306, 29.0787) knots 0 0 0 1 2 2 2
  line L1445 (-10.0975, 29.6118) -> (-10.0975, 29.391) construction
  line L1446 (-10.0975, 29.391) -> (-10.4098, 29.0787) construction
  line L1447 (-10.4098, 29.0787) -> (-10.6306, 29.0787) construction
  line L1448 (-10.6306, 29.0787) -> (-10.8982, 29.0787)
  spline S440 degree 2 poles (-10.8982, 29.0787) (-11.1168, 29.0787) (-11.4312, 29.391) (-11.4312, 29.6118) knots 0 0 0 1 2 2 2
  line L1449 (-10.8982, 29.0787) -> (-11.1168, 29.0787) construction
  line L1450 (-11.1168, 29.0787) -> (-11.4312, 29.391) construction
  line L1451 (-11.4312, 29.391) -> (-11.4312, 29.6118) construction
  line L1452 (-11.4312, 29.6118) -> (-11.4312, 31.2689)
  spline S441 degree 2 poles (-11.4312, 31.2689) (-11.4312, 31.4941) (-11.2818, 31.628) knots 0 0 0 1 1 1
  line L1453 (-11.4312, 31.2689) -> (-11.4312, 31.4941) construction
  line L1454 (-11.4312, 31.4941) -> (-11.2818, 31.628) construction
  spline S442 degree 2 poles (-11.2818, 31.628) (-11.1458, 31.7484) (-10.9473, 31.7484) knots 0 0 0 1 1 1
  line L1455 (-11.2818, 31.628) -> (-11.1458, 31.7484) construction
  line L1456 (-11.1458, 31.7484) -> (-10.9473, 31.7484) construction
  spline S443 degree 2 poles (-10.9473, 31.7484) (-10.7532, 31.7484) (-10.6194, 31.6302) knots 0 0 0 1 1 1
  line L1457 (-10.9473, 31.7484) -> (-10.7532, 31.7484) construction
  line L1458 (-10.7532, 31.7484) -> (-10.6194, 31.6302) construction
  spline S444 degree 2 poles (-10.6194, 31.6302) (-10.47, 31.4964) (-10.47, 31.2711) knots 0 0 0 1 1 1
  line L1459 (-10.6194, 31.6302) -> (-10.47, 31.4964) construction
  line L1460 (-10.47, 31.4964) -> (-10.47, 31.2711) construction
  spline S445 degree 2 poles (-10.47, 31.2711) (-10.47, 31.0458) (-10.6306, 30.9388) knots 0 0 0 1 1 1
  line L1461 (-10.47, 31.2711) -> (-10.47, 31.0458) construction
  line L1462 (-10.47, 31.0458) -> (-10.6306, 30.9388) construction
  spline S446 degree 2 poles (-10.6306, 30.9388) (-10.3719, 30.9388) (-10.2291, 30.7871) knots 0 0 0 1 1 1
  line L1463 (-10.6306, 30.9388) -> (-10.3719, 30.9388) construction
  line L1464 (-10.3719, 30.9388) -> (-10.2291, 30.7871) construction
  spline S447 degree 2 poles (-12.4973, 29.0787) (-12.7159, 29.0787) (-13.0326, 29.391) (-13.0326, 29.6118) knots 0 0 0 1 2 2 2
  line L1465 (-12.4973, 29.0787) -> (-12.7159, 29.0787) construction
  line L1466 (-12.7159, 29.0787) -> (-13.0326, 29.391) construction
  line L1467 (-13.0326, 29.391) -> (-13.0326, 29.6118) construction
  line L1468 (-13.0326, 29.6118) -> (-13.0326, 30.4147)
  spline S448 degree 2 poles (-13.0326, 30.4147) (-13.0326, 30.6355) (-12.7159, 30.9477) (-12.4973, 30.9477) knots 0 0 0 1 2 2 2
  line L1469 (-13.0326, 30.4147) -> (-13.0326, 30.6355) construction
  line L1470 (-13.0326, 30.6355) -> (-12.7159, 30.9477) construction
  line L1471 (-12.7159, 30.9477) -> (-12.4973, 30.9477) construction
  line L1472 (-12.4973, 30.9477) -> (-12.0981, 30.9477)
  spline S449 degree 2 poles (-12.0981, 30.9477) (-11.9643, 30.9477) (-11.9643, 30.8139) knots 0 0 0 1 1 1
  line L1473 (-12.0981, 30.9477) -> (-11.9643, 30.9477) construction
  line L1474 (-11.9643, 30.9477) -> (-11.9643, 30.8139) construction
  spline S450 degree 2 poles (-11.9643, 30.8139) (-11.9643, 30.6801) (-12.0981, 30.6801) knots 0 0 0 1 1 1
  line L1475 (-11.9643, 30.8139) -> (-11.9643, 30.6801) construction
  line L1476 (-11.9643, 30.6801) -> (-12.0981, 30.6801) construction
  line L1477 (-12.0981, 30.6801) -> (-12.4973, 30.6801)
  spline S451 degree 2 poles (-12.4973, 30.6801) (-12.6066, 30.6801) (-12.7649, 30.5217) (-12.7649, 30.4124) knots 0 0 0 1 2 2 2
  line L1478 (-12.4973, 30.6801) -> (-12.6066, 30.6801) construction
  line L1479 (-12.6066, 30.6801) -> (-12.7649, 30.5217) construction
  line L1480 (-12.7649, 30.5217) -> (-12.7649, 30.4124) construction
  line L1481 (-12.7649, 30.4124) -> (-12.7649, 29.614)
  spline S452 degree 2 poles (-12.7649, 29.614) (-12.7649, 29.5047) (-12.6066, 29.3464) (-12.4973, 29.3464) knots 0 0 0 1 2 2 2
  line L1482 (-12.7649, 29.614) -> (-12.7649, 29.5047) construction
  line L1483 (-12.7649, 29.5047) -> (-12.6066, 29.3464) construction
  line L1484 (-12.6066, 29.3464) -> (-12.4973, 29.3464) construction
  line L1485 (-12.4973, 29.3464) -> (-12.0981, 29.3464)
  spline S453 degree 2 poles (-12.0981, 29.3464) (-11.9643, 29.3464) (-11.9643, 29.2126) knots 0 0 0 1 1 1
  line L1486 (-12.0981, 29.3464) -> (-11.9643, 29.3464) construction
  line L1487 (-11.9643, 29.3464) -> (-11.9643, 29.2126) construction
  spline S454 degree 2 poles (-11.9643, 29.2126) (-11.9643, 29.0787) (-12.0981, 29.0787) knots 0 0 0 1 1 1
  line L1488 (-11.9643, 29.2126) -> (-11.9643, 29.0787) construction
  line L1489 (-11.9643, 29.0787) -> (-12.0981, 29.0787) construction
  line L1490 (-12.0981, 29.0787) -> (-12.4973, 29.0787)
  spline S455 degree 2 poles (-9.0292, 30.6801) (-9.1541, 30.6801) (-9.2946, 30.524) (-9.2946, 30.4147) knots 0 0 0 1 2 2 2
  line L1491 (-9.0292, 30.6801) -> (-9.1541, 30.6801) construction
  line L1492 (-9.1541, 30.6801) -> (-9.2946, 30.524) construction
  line L1493 (-9.2946, 30.524) -> (-9.2946, 30.4147) construction
  spline S456 degree 2 poles (-9.2946, 30.4147) (-9.2946, 30.3054) (-9.2277, 30.2296) knots 0 0 0 1 1 1
  line L1494 (-9.2946, 30.4147) -> (-9.2946, 30.3054) construction
  line L1495 (-9.2946, 30.3054) -> (-9.2277, 30.2296) construction
  spline S457 degree 2 poles (-9.2277, 30.2296) (-9.1541, 30.147) (-9.0292, 30.147) knots 0 0 0 1 1 1
  line L1496 (-9.2277, 30.2296) -> (-9.1541, 30.147) construction
  line L1497 (-9.1541, 30.147) -> (-9.0292, 30.147) construction
  spline S458 degree 2 poles (-9.3169, 29.139) (-9.3571, 29.0765) (-9.424, 29.0765) knots 0 0 0 1 1 1
  line L1498 (-9.3169, 29.139) -> (-9.3571, 29.0765) construction